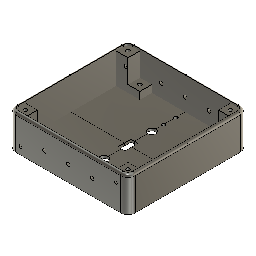
main_case (Autodesk Fusion 360 design; units mm, degrees)
Autodesk Fusion 360 part; units mm, degrees
sketch "Skizze1" plane through (0, 0, 0) normal (0, 0, 1) x (1, 0, 0)
  line L0 (0, 0) -> (50, 0)
  line L1 (50, 0) -> (50, 50)
  line L2 (50, 50) -> (0, 50)
  line L3 (0, 50) -> (0, 0)
  dimension "d1" = 50
  dimension "d2" = 50
  constraint horizontal L0
  constraint vertical L1
  constraint horizontal L2
  constraint vertical L3
  constraint coincident L0.start L3.end
  measures "d1" distance of L0.start L0.end
  measures "d2" distance of L0.end L1.end
extrude "Extrusion1" add sketch "Skizze1" along normal blind 29 makes body 1
sketch "Skizze2" plane through (0, 0, 29) normal (0, 0, 1) x (-1, 0, 0)
  line L0 (0, -50) -> (0, 0)
  line L1 (0, 0) -> (-50, 0)
  line L2 (-50, 0) -> (-50, -50)
  line L3 (-50, -50) -> (0, -50)
  line L4 (0, 0) -> (-48, 0)
  line L5 (-48, 0) -> (-48, -48)
  line L6 (-48, -48) -> (0, -48)
  line L7 (0, -48) -> (0, 0)
  dimension "d5" = 2
  dimension "d6" = 2
  constraint horizontal L4
  constraint vertical L5
  constraint horizontal L6
  constraint vertical L7
  constraint coincident L0.end L1.start
  measures "d5" distance of L2 L5
  measures "d6" distance of L3 L6
extrude "Extrusion2" cut sketch "Skizze2" against normal blind 27 contours L0 L1 L4 L5 L6 L7 bodies 1
sketch "Skizze3" plane through (0, 0, 2) normal (0, 0, 1) x (-1, 0, 0)
  line L0 (0, -48) -> (0, 0)
  line L1 (0, 0) -> (-48, 0)
  line L2 (-48, 0) -> (-48, -48)
  line L3 (-48, -48) -> (0, -48)
  line L4 (-48, -48) -> (-38, -48)
  line L5 (-38, -48) -> (-38, -38)
  line L6 (-38, -38) -> (-48, -38)
  line L7 (-48, -38) -> (-48, -48)
  dimension "d9" = 10
  dimension "d10" = 10
  constraint horizontal L4
  constraint vertical L5
  constraint horizontal L6
  constraint vertical L7
  constraint coincident L2.end L3.start
  measures "d9" distance of L5.end L6.end
  measures "d10" distance of L4.end L5.end
extrude "Extrusion3" add sketch "Skizze3" along normal blind 25.4 contours L2 L3 L4 L5 L6 L7 bodies 1
sketch "Skizze4" plane through (0, 0, 2) normal (0, 0, 1) x (-1, 0, 0)
  line L0 (-48, -38) -> (-38, -38)
  line L1 (-38, -38) -> (-38, -48)
  line L2 (-38, -48) -> (0, -48)
  line L3 (0, -48) -> (0, 0)
  line L4 (0, 0) -> (-48, 0)
  line L5 (-48, 0) -> (-48, -38)
  line L6 (0, 0) -> (-3.04, 0)
  line L7 (-3.04, 0) -> (-3.04, -5.58)
  line L8 (-3.04, -5.58) -> (0, -5.58)
  line L9 (0, -5.58) -> (0, 0)
  dimension "d13" = 3.04
  dimension "d14" = 5.58
  constraint horizontal L6
  constraint vertical L7
  constraint horizontal L8
  constraint vertical L9
  constraint coincident L3.end L4.start
  measures "d13" distance of L3.end L6.end
  measures "d14" distance of L6.end L7.end
extrude "Extrusion4" cut sketch "Skizze4" against normal through all contours L3 L4 L6 L7 L8 L9 bodies 1
sketch "Skizze5" plane through (0, 0, 2) normal (0, 0, 1) x (-1, 0, 0)
  line L0 (0, -5.58) -> (-3.04, -5.58)
  line L1 (-3.04, -5.58) -> (-3.04, 0)
  line L2 (-3.04, 0) -> (-48, 0)
  line L3 (-48, 0) -> (-48, -38)
  line L4 (-48, -38) -> (-38, -38)
  line L5 (-38, -38) -> (-38, -48)
  line L6 (-38, -48) -> (0, -48)
  line L7 (0, -48) -> (0, -5.58)
  point P0 (0, -40)
  dimension "d17" = 40
  constraint coincident L7 P0
  measures "d17" distance of L2 P0
hole "Bohrung1" at (0, 40, 2) direction (0, 0, -1) diameter 3.2 depth 10 tip angle 118 bodies 1
sketch "Skizze6" plane through (0, 0, 27.4) normal (0, 0, 1) x (-1, 0, 0)
  line L0 (-38, -48) -> (-38, -38)
  line L1 (-38, -38) -> (-48, -38)
  line L2 (-48, -38) -> (-48, -48)
  line L3 (-48, -48) -> (-38, -48)
  point P0 (-43, -43)
hole "Bohrung2" at (43, 43, 27.4) direction (0, 0, -1) diameter 3.2 end through all bodies 1
sketch "Skizze7" plane through (0, 0, 0) normal (0, 0, -1) x (1, 0, 0)
  line L0 (0, -41.6) -> (0, -50)
  line L1 (0, -50) -> (50, -50)
  line L2 (50, -50) -> (50, 0)
  line L3 (50, 0) -> (3.04, 0)
  line L4 (41.3257, -40.1) -> (39.6514, -43)
  line L5 (39.6514, -43) -> (41.3257, -45.9)
  line L6 (41.3257, -45.9) -> (44.6743, -45.9)
  line L7 (44.6743, -45.9) -> (46.3486, -43)
  line L8 (46.3486, -43) -> (44.6743, -40.1)
  line L9 (44.6743, -40.1) -> (41.3257, -40.1)
  circle A0 centre (43, -43) radius 1.6
  arc A1 (0, -41.6) -> (0, -38.4) centre (0, -40) ccw
  line L10 (3.04, 0) -> (3.04, -5.58)
  line L11 (3.04, -5.58) -> (0, -5.58)
  line L12 (0, -5.58) -> (0, -38.4)
  point P0 (43, -43)
  dimension "d26" = 5.8
  constraint parallel L1 L6
  constraint coincident P0 A0.centre
  measures "d26" distance of L6 L9
extrude "Extrusion5" cut sketch "Skizze7" against normal blind 12.5 contours L4 L5 L6 L7 L8 L9 | A0 bodies 1
fillet "Abrundung1" radius 4 1 edges at (48, 48, 28.2) on bodies 1
fillet "Abrundung2" radius 6 1 edges at (50, 50, 14.5) on bodies 1
sketch "Skizze8" plane through (0, 0, 2) normal (0, 0, 1) x (-1, 0, 0)
  arc A0 (0, -38.4) -> (0, -41.6) centre (0, -40) ccw
  line L0 (0, -38.4) -> (0, -5.58)
  line L1 (0, -5.58) -> (-3.04, -5.58)
  line L2 (-3.04, -5.58) -> (-3.04, 0)
  line L3 (-3.04, 0) -> (-48, 0)
  line L4 (-48, 0) -> (-48, -38)
  line L5 (-48, -38) -> (-38, -38)
  line L6 (-38, -38) -> (-38, -48)
  line L7 (-38, -48) -> (0, -48)
  line L8 (0, -48) -> (0, -41.6)
  line L9 (-38, -38) -> (-28, -38)
  line L10 (-28, -38) -> (-28, -48)
  line L11 (-28, -48) -> (-38, -48)
  line L12 (-38, -48) -> (-38, -38)
  dimension "d35" = 10
  dimension "d36" = 10
  constraint horizontal L9
  constraint vertical L10
  constraint horizontal L11
  constraint vertical L12
  constraint coincident L7 L10.end
  constraint coincident L6 L5.end
  measures "d35" distance of L5.end L9.end
  measures "d36" distance of L9.end L10.end
extrude "Extrusion6" add sketch "Skizze8" along normal blind 6 contours L6 L7 L9 L10 L11 L12 bodies 1
sketch "Skizze9" plane through (0, 0, 8) normal (0, 0, 1) x (-1, 0, 0)
  line L0 (-38, -48) -> (-28, -48)
  line L1 (-28, -48) -> (-28, -38)
  line L2 (-28, -38) -> (-38, -38)
  line L3 (-38, -38) -> (-38, -48)
  point P0 (-33, -43)
  dimension "d39" = 5
  dimension "d40" = 5
  measures "d39" distance of L0 P0
  measures "d40" distance of L3 P0
hole "Bohrung3" at (33, 43, 8) direction (0, 0, -1) diameter 3.2 end through all bodies 1
sketch "Skizze10" plane through (0, 0, 0) normal (0, 0, -1) x (1, 0, 0)
  arc A0 (44, -50) -> (50, -44) centre (44, -44) ccw
  line L0 (50, -44) -> (50, 0)
  line L1 (50, 0) -> (3.04, 0)
  line L2 (0, -5.58) -> (0, -38.4)
  line L3 (0, -50) -> (44, -50)
  line L4 (31.3257, -40.1) -> (29.6514, -43)
  line L5 (29.6514, -43) -> (31.3257, -45.9)
  line L6 (31.3257, -45.9) -> (34.6743, -45.9)
  line L7 (34.6743, -45.9) -> (36.3486, -43)
  line L8 (36.3486, -43) -> (34.6743, -40.1)
  line L9 (34.6743, -40.1) -> (31.3257, -40.1)
  circle A1 centre (33, -43) radius 1.6
  line L10 (44.6743, -45.9) -> (41.3257, -45.9)
  line L11 (41.3257, -45.9) -> (39.6514, -43)
  line L12 (39.6514, -43) -> (41.3257, -40.1)
  line L13 (41.3257, -40.1) -> (44.6743, -40.1)
  line L14 (44.6743, -40.1) -> (46.3486, -43)
  line L15 (46.3486, -43) -> (44.6743, -45.9)
  line L16 (3.04, 0) -> (3.04, -5.58)
  line L17 (3.04, -5.58) -> (0, -5.58)
  arc A2 (0, -41.6) -> (0, -38.4) centre (0, -40) ccw
  line L18 (0, -41.6) -> (0, -50)
  point P0 (33, -43)
  dimension "d44" = 5.8
  constraint parallel L3 L6
  measures "d44" distance of L6 L9
extrude "Extrusion7" cut sketch "Skizze10" against normal blind 4 contours L4 L5 L6 L7 L8 L9 | A1 bodies 1
fillet "Abrundung4" radius 2 3 edges at (50, 22, 29) (48.2426, 48.2426, 29) (22, 50, 29) on bodies 1
sketch "Skizze14" plane through (0, 0, 2) normal (0, 0, 1) x (-1, 0, 0)
  line L0 (-28, -38) -> (-28, -48)
  line L1 (-28, -48) -> (0, -48)
  line L2 (0, -48) -> (0, -41.6)
  arc A0 (0, -38.4) -> (0, -41.6) centre (0, -40) ccw
  line L3 (0, -38.4) -> (0, -5.58)
  line L4 (0, -5.58) -> (-3.04, -5.58)
  line L5 (-3.04, -5.58) -> (-3.04, 0)
  line L6 (-3.04, 0) -> (-48, 0)
  line L7 (-48, 0) -> (-48, -38)
  line L8 (-48, -38) -> (-28, -38)
  point P0 (0, -20)
  dimension "d79" = 20
  constraint coincident L3 P0
  measures "d79" distance of L6 P0
hole "Bohrung7" at (0, 20, 2) direction (0, 0, -1) diameter 7 end through all bodies 1
mirror "Spiegeln1" about plane through (0, 0, 0) normal (1, 0, 0) of "Extrusion1", "Extrusion2", "Extrusion3", "Extrusion4", "Bohrung1", "Bohrung2", "Extrusion5", "Abrundung1", "Abrundung2", "Extrusion6", "Bohrung3", "Extrusion7", "Abrundung4", "Bohrung7" makes body 2
mirror "Spiegeln2" about plane through (0, 0, 0) normal (0, 1, 0) of "Extrusion1", "Extrusion2", "Extrusion3", "Extrusion4", "Bohrung1", "Bohrung2", "Extrusion5", "Abrundung1", "Abrundung2", "Extrusion6", "Bohrung3", "Extrusion7", "Abrundung4", "Bohrung7", "Spiegeln1" makes body 3 at (28.246, -19.7737, 0) makes body 4 at (-28.246, -19.7737, 0)
sketch "Skizze11" plane through (0, -50, 0) normal (0, -1, 0) x (1, 0, 0)
  line L0 (0, 27) -> (-44, 27)
  line L1 (-44, 27) -> (-44, 0)
  line L2 (-44, 0) -> (0, 0)
  line L3 (0, 0) -> (0, 27)
  line L4 (44, 0) -> (0, 0)
  point P0 (0, 13)
  point P1 (20, 13)
  point P2 (-20, 13)
  dimension "d56" = 20
  dimension "d57" = 20
  dimension "d58" = 13
  dimension "d59" = 27
  dimension "d60" = 13
  dimension "d61" = 13
  constraint coincident L3 P0
  measures "d56" distance of P0 P1
  measures "d57" distance of P0 P2
  measures "d58" distance of L2 P2
  measures "d59" distance of L0 L2
  measures "d60" distance of P0 L4
  measures "d61" distance of P1 L4
hole "Bohrung4" at (20, -50, 13) at (0, -50, 13) at (-20, -50, 13) direction (0, 1, 0) diameter 3.2 end through all bodies 1 2 3 4
sketch "Skizze12" plane through (0, -50, 0) normal (0, -1, 0) x (1, 0, 0)
  arc A0 (0, 14.6) -> (0, 11.4) centre (0, 13) ccw
  line L0 (0, 14.6) -> (0, 27)
  line L1 (0, 27) -> (-44, 27)
  line L2 (-44, 27) -> (-44, 0)
  line L3 (-44, 0) -> (0, 0)
  line L4 (0, 0) -> (0, 11.4)
  circle A1 centre (-20, 13) radius 1.6
  circle A2 centre (20, 13) radius 1.6
  point P0 (40, 20)
  point P1 (-40, 6)
  dimension "d65" = 40
  dimension "d66" = 40
  dimension "d67" = 7
  dimension "d68" = 7
  measures "d65" horizontal distance of A0.centre P1
  measures "d66" horizontal distance of A0.centre P0
  measures "d67" vertical distance of P0 A2.centre
  measures "d68" vertical distance of A1.centre P1
hole "Bohrung5" at (-40, -50, 6) at (40, -50, 20) direction (0, 1, 0) diameter 2.5 depth 20 tip angle 118 bodies 3 4
sketch "Skizze13" plane through (0, 50, 0) normal (0, 1, 0) x (-1, 0, 0)
  arc A0 (0, 11.4) -> (0, 14.6) centre (0, 13) ccw
  line L0 (0, 11.4) -> (0, 0)
  line L1 (0, 0) -> (44, 0)
  line L2 (44, 0) -> (44, 27)
  line L3 (44, 27) -> (0, 27)
  line L4 (0, 27) -> (0, 14.6)
  circle A1 centre (20, 13) radius 1.6
  circle A2 centre (-20, 13) radius 1.6
  point P0 (40, 20)
  point P1 (-40, 6)
  dimension "d72" = 40
  dimension "d73" = 7
  dimension "d74" = 40
  dimension "d75" = 7
  measures "d72" horizontal distance of A0.centre P1
  measures "d73" vertical distance of P1 A2.centre
  measures "d74" horizontal distance of A0.centre P0
  measures "d75" vertical distance of A1.centre P0
hole "Bohrung6" at (-40, 50, 20) at (40, 50, 6) direction (0, -1, 0) diameter 2.5 depth 20 tip angle 118 bodies 1 2
sketch "Skizze15" plane through (0, 0, 2) normal (0, 0, 1) x (-1, 0, 0)
  arc A0 (0, -16.5) -> (0, -23.5) centre (0, -20) ccw
  line L0 (0, -16.5) -> (0, -5.58)
  line L1 (0, -5.58) -> (-3.04, -5.58)
  line L2 (-3.04, -5.58) -> (-3.04, 0)
  line L3 (-3.04, 0) -> (-48, 0)
  line L4 (-48, 0) -> (-48, -38)
  line L5 (-48, -38) -> (-28, -38)
  line L6 (-28, -38) -> (-28, -48)
  line L7 (-28, -48) -> (0, -48)
  line L8 (0, -48) -> (0, -41.6)
  arc A1 (0, -38.4) -> (0, -41.6) centre (0, -40) ccw
  line L9 (0, -38.4) -> (0, -23.5)
  point P0 (0, -30)
  dimension "d83" = 30
  constraint coincident L9 P0
  measures "d83" distance of origin P0
hole "Bohrung8" at (0, 30, 2) direction (0, 0, -1) diameter 3.2 end through all bodies 1 2
equation "d3 = height"
equation "d7 = -height + 2 mm"
equation "d11 = height - 2 mm - 1.6 mm"
equation "d13 = 2.54 mm + 0.5 mm"
equation "d14 = ( 2.54 * 2 ) * 1 mm + 0.5 mm"
equation "height = 29 mm"
equation "d58 = 26.00 mm / 2"
